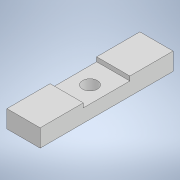
# Autodesk Inventor part: Belt Clamp
Saved by Autodesk Inventor 2022 (Build 260153000, 153)
## iProperties
Created: 2023-01-05
Part Number: Belt Clamp
Material: Generic
Document SubType Name: Modeling
Designer: Gaming
Density: 1 g/cm^3
Appearance: Default
Author: Gaming
Autodesk Inventor part; units mm, degrees
ref_plane "YZ Plane" through (0, 0, 0) normal (1, 0, 0) x (0, 1, 0)
ref_plane "XZ Plane" through (0, 0, 0) normal (0, 1, 0) x (-1, 0, 0)
ref_plane "XY Plane" through (0, 0, 0) normal (0, 0, 1) x (1, 0, 0)
sketch "Sketch1" plane through (0, 0, 0) normal (0, 1, 0) x (-1, 0, 0)
  line L0 (5, 20) -> (-5, 20)
  line L1 (-5, 20) -> (-5, -20)
  line L2 (-5, -20) -> (5, -20)
  line L3 (5, -20) -> (5, 20)
  point P0 (0, 0)
  point P1 (0, -20)
  point P2 (-5, 0)
  dimension "d0" = 10
  dimension "d1" = 40
  constraints: 8 end point, 2 midpoint, 2 parallel, 1 horizontal, 1 horizontal alignment, 1 perpendicular, 1 vertical alignment
  measures "d0" distance of L2.end L1.end
  measures "d1" distance of L1.end L0.end
extrude "Extrusion1" add sketch "Sketch1" along normal blind 4
sketch "Sketch2" plane through (0, 4, 0) normal (0, 1, 0) x (1, 0, 0)
  line L0 (-5, 20) -> (-5, -20) projected
  line L1 (5, -20) -> (5, 20) projected
  line L2 (-5, -20) -> (5, -20)
  line L3 (5, -20) -> (5, -7)
  line L4 (5, -7) -> (-5, -7)
  line L5 (-5, -7) -> (-5, -20)
  line L6 (5, 20) -> (-5, 20) projected
  line L7 (-5, 20) -> (5, 20)
  line L8 (5, 20) -> (5, 7)
  line L9 (5, 7) -> (-5, 7)
  line L10 (-5, 7) -> (-5, 20)
  point P0 (0, 0)
  dimension "d4" = 13
  dimension "d5" = 13
  constraints: 16 end point, 4 parallel, 2 horizontal, 2 perpendicular, 2 point on line
  measures "d4" distance of L0.start L9.end
  measures "d5" distance of L0.end L4.end
extrude "Extrusion2" add sketch "Sketch2" along normal blind 1.3 contours L6 L1 L9 L0 | L4 L1 L2 L0
sketch "Sketch3" plane through (0, 4, 0) normal (0, 1, 0) x (1, 0, 0)
  point P0 (0, 0)
  point P1 (0, 0)
  constraints: 1 coincident
hole "Hole1" at (0, 4, 0) direction (0, -1, 0) diameter 4.5 end through all
body "Solid1"
